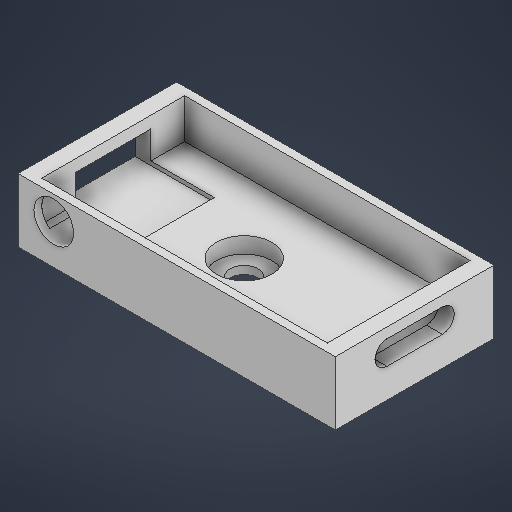
# Autodesk Inventor part: elektronika
Saved by Autodesk Inventor 2027 (Build 310192060, 192F)
## iProperties
Created: 2026-05-15
Part Number: elektronika
Material: Ogólny
Document SubType Name: Modeling
Designer: User
Density: 1 g/cm^3
Appearance: Domyślna
Author: User
Autodesk Inventor part; units mm, degrees
ref_plane "YZ Plane" through (0, 0, 0) normal (1, 0, 0) x (0, 1, 0)
ref_plane "XZ Plane" through (0, 0, 0) normal (0, 1, 0) x (-1, 0, 0)
ref_plane "XY Plane" through (0, 0, 0) normal (0, 0, 1) x (1, 0, 0)
sketch "Szkic1" plane through (0, 0, 0) normal (0, 1, 0) x (-1, 0, 0)
  circle A0 centre (0, 0) radius 1.75
  line L0 (18.5, 10) -> (-21.5, 10)
  line L1 (-21.5, 10) -> (-21.5, -10)
  line L2 (-21.5, -10) -> (18.5, -10)
  line L3 (18.5, -10) -> (18.5, 10)
  line L4 (-19.5, 9) -> (16.5, 9)
  line L5 (16.5, 9) -> (16.5, -9)
  line L6 (16.5, -9) -> (-19.5, -9)
  line L7 (-19.5, -9) -> (-19.5, 9)
  dimension "d0" = 3.5
  dimension "d1" = 20
  dimension "d2" = 40
  dimension "d3" = 36
  dimension "d4" = 18
  dimension "d9" = 16.5
  dimension "d10" = 2
  constraints: 16 end point, 4 parallel, 2 horizontal, 2 perpendicular, 1 centre point, 1 coincident
  measures "d0" diameter of A0
  measures "d1" distance of L1.end L0.end
  measures "d2" distance of L0.start L0.end
  measures "d3" distance of L5.end L6.end
  measures "d4" distance of L4.end L5.end
  measures "d9" distance from line of L5 A0.centre
  measures "d10" distance between parallel lines of L3 L5
extrude "Wyciągnięcie proste1" add sketch "Szkic1" along normal blind 6 contours L3 L2 L1 L0
extrude "Wyciągnięcie proste2" add sketch "Szkic1" along normal blind 1 and the other way blind 2 contours L3 L2 L1 L0 | L4 L5 L6 L7
sketch "Szkic2" plane through (21.5, 0, 10) normal (1, 0, 0) x (0, 0, -1)
  line L0 (10, 0) -> (10, 3.2)
  line L1 (10, 0) -> (13.2, 0) construction
  line L2 (6.5, 3.2) -> (13.5, 3.2) construction
  line L3 (6.5, 1.7) -> (13.5, 1.7)
  line L4 (13.5, 4.7) -> (6.5, 4.7)
  arc A0 (6.5, 4.7) -> (6.5, 1.7) centre (6.5, 3.2) ccw
  arc A1 (13.5, 1.7) -> (13.5, 4.7) centre (13.5, 3.2) ccw
  dimension "d11" = 3.2
  dimension "d12" = 90
  dimension "d13" = 3.5
  dimension "d14" = 3
  constraints: 12 end point, 4 point on circle, 4 tangent, 2 centre point, 2 horizontal, 1 midpoint, 1 parallel, 1 perpendicular, 1 vertical
  measures "d11" distance of L0.start L0.end
  measures "d12" angle of L1 L0
  measures "d13" distance of L0.end L2.end
  measures "d14" diameter of A1
extrude "Wyciągnięcie proste3" cut sketch "Szkic2" against normal blind 10
sketch "Szkic3" plane through (-18.5, 0, -10) normal (-1, 0, 0) x (0, 0, 1)
  line L0 (10, 0) -> (10, 2.5)
  line L1 (10, 0) -> (12.5, 0) construction
  line L2 (5.25, 4.5) -> (14.75, 4.5)
  line L3 (14.75, 4.5) -> (14.75, 0.5)
  line L4 (14.75, 0.5) -> (5.25, 0.5)
  line L5 (5.25, 0.5) -> (5.25, 4.5)
  line L6 (5.25, 4.5) -> (14.75, 0.5) construction
  line L7 (14.75, 4.5) -> (5.25, 0.5) construction
  dimension "d17" = 2.5
  dimension "d18" = 90
  dimension "d19" = 9.5
  dimension "d20" = 4
  constraints: 16 end point, 2 horizontal, 2 midpoint, 2 parallel, 2 perpendicular, 1 vertical
  measures "d17" distance of L0.start L0.end
  measures "d18" angle of L1 L0
  measures "d19" distance of L3.end L4.end
  measures "d20" distance of L2.end L3.end
extrude "Wyciągnięcie proste4" cut sketch "Szkic3" against normal blind 10
sketch "Szkic4" plane through (0, 1, 0) normal (0, 1, 0) x (1, 0, 0)
  circle A0 centre (0, 0) radius 1.75 projected
  circle A1 centre (0, 0) radius 3.5
  dimension "d23" = 7
  constraints: 1 centre point, 1 coincident
  measures "d23" diameter of A1
extrude "Wyciągnięcie proste5" cut sketch "Szkic4" against normal blind 2
sketch "Szkic5" plane through (-18.5, 6, 10) normal (0, 0, 1) x (1, 0, 0)
  line L0 (2, -5) -> (2, 0) projected
  line L1 (2, -5) -> (2, 0)
  line L2 (2, 0) -> (2, -5)
  line L3 (2, -5) -> (2, -5.5)
  line L4 (0, -5.5) -> (10, -5.5) projected
  line L5 (2, -5.5) -> (7, -5.5)
  circle A0 centre (4.5, -3) radius 2.5
  point P0 (18.5, -6)
  dimension "d28" = 5
  dimension "d29" = 5
  dimension "d32" = 2.5
  dimension "d33" = 2.5
  constraints: 8 end point, 2 collinear, 2 point on line, 1 centre point, 1 vertical
  measures "d28" distance of L3.end L5.end
  measures "d29" diameter of A0
  measures "d32" distance from line of L0 A0.centre
  measures "d33" distance from line of L4 A0.centre
extrude "Wyciągnięcie proste6" cut sketch "Szkic5" against normal blind 10 contours A0
